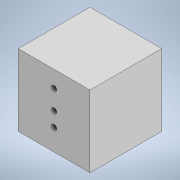
# Autodesk Inventor part: HammerPod
Saved by Autodesk Inventor 2020 (Build 240168000, 168)
## iProperties
Created: 2019-11-18
Part Number: HammerPod
Material: 일반
Document SubType Name: Modeling
Designer: Knowblesse
Density: 1 g/cm^3
Appearance: 기본값
Author: Knowblesse
## iProperties of the stored document _3D 인쇄.ipt
Created: 2019-11-18
Part Number: _3D 인쇄
Material: 일반
Document SubType Name: Modeling
Designer: Knowblesse
Density: 1 g/cm^3
Appearance: 기본값
Author: Knowblesse
Autodesk Inventor part; units mm, degrees
ref_plane "YZ Plane" through (0, 0, 0) normal (1, 0, 0) x (0, 1, 0)
ref_plane "XZ Plane" through (0, 0, 0) normal (0, 1, 0) x (-1, 0, 0)
ref_plane "XY Plane" through (0, 0, 0) normal (0, 0, 1) x (1, 0, 0)
sketch "스케치1" plane through (0, 0, 0) normal (0, 0, 1) x (1, 0, 0)
  line L0 (0, 0) -> (20, 0)
  line L1 (20, 0) -> (20, 20)
  line L2 (20, 20) -> (0, 20)
  line L3 (0, 20) -> (0, 0)
  dimension "d0" = 20
  dimension "d1" = 20
  constraints: 8 end point, 2 parallel, 1 horizontal, 1 perpendicular
  measures "d0" distance of L2.end L1.end
  measures "d1" distance of L1.end L0.end
extrude "돌출1" add sketch "스케치1" along normal blind 20
sketch "스케치2" plane through (0, 0, 20) normal (0, 0, 1) x (1, 0, 0)
  line L0 (0, 0) -> (20, 0) projected
  line L1 (20, 0) -> (20, 20) projected
  line L2 (20, 20) -> (0, 20) projected
  line L3 (0, 20) -> (0, 0) projected
  line L4 (20, 0) -> (20, 20) construction
  line L5 (20, 10) -> (0, 10) construction
  line L6 (0, 20) -> (0, 0) construction
  line L7 (0, 0) -> (20, 0) construction
  line L8 (10, 0) -> (10, 20) construction
  line L9 (20, 20) -> (0, 20) construction
  point P0 (10, 10)
  point P1 (10, 6)
  point P2 (10, 10)
  point P3 (10, 10)
  point P4 (10, 15.4)
  dimension "d11" = 4
  dimension "d12" = 5.4
  constraints: 6 midpoint, 4 end point, 1 coincident, 1 point on line, 1 vertical alignment
  measures "d11" distance of point (10, 6) point (10, 10)
  measures "d12" distance of point (10, 10) point (10, 15.4)
hole "구멍1" at (10, 10, 20) at (10, 15.4, 20) at (10, 6, 20) direction (0, 0, -1) diameter 1.5 end through all
